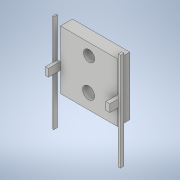
# Autodesk Inventor part: filter wheel
Saved by Autodesk Inventor 2021 (Build 250183000, 183)
## iProperties
Created: 2019-03-06
Part Number: filter wheel
Material: Generic
Document SubType Name: Modeling
Designer: Saumya
Density: 1 g/cm^3
Appearance: Default
Author: Saumya
Autodesk Inventor part; units mm, degrees
ref_plane "YZ Plane" through (0, 0, 0) normal (1, 0, 0) x (0, 1, 0)
ref_plane "XZ Plane" through (0, 0, 0) normal (0, 1, 0) x (-1, 0, 0)
ref_plane "XY Plane" through (0, 0, 0) normal (0, 0, 1) x (1, 0, 0)
sketch "Sketch1" plane through (0, 0, 0) normal (0, 0, 1) x (1, 0, 0)
  circle A0 centre (101.883, 74.9428) radius 12.7
  line L0 (42.2826, 167.437) -> (163.579, 167.437)
  line L1 (163.579, 167.437) -> (163.579, 43.6004)
  line L2 (163.579, 43.6004) -> (42.2826, 43.6004)
  line L3 (42.2826, 43.6004) -> (42.2826, 167.437)
  circle A1 centre (102.9308, 142.9872) radius 11.691
  line L4 (42.2826, 116.6323) -> (31.1691, 116.6323)
  line L5 (31.1691, 116.6323) -> (31.1691, 96.9454)
  line L6 (31.1691, 96.9454) -> (42.2826, 96.9454)
  line L7 (42.2826, 96.9454) -> (42.2826, 116.6323)
  line L8 (163.579, 116.6323) -> (174.375, 116.6323)
  line L9 (174.375, 116.6323) -> (174.375, 96.9454)
  line L10 (174.375, 96.9454) -> (163.579, 96.9454)
  line L11 (163.579, 96.9454) -> (163.579, 116.6323)
  line L12 (31.1691, 126.4757) -> (23.2309, 126.4757)
  line L13 (23.2309, 126.4757) -> (23.2309, 0)
  line L14 (23.2309, 0) -> (31.1691, 0)
  line L15 (31.1691, 0) -> (31.1691, 126.4757)
  line L16 (174.375, 126.4757) -> (184.536, 126.4757)
  line L17 (184.536, 126.4757) -> (184.536, 0)
  line L18 (184.536, 0) -> (174.375, 0)
  line L19 (174.375, 0) -> (174.375, 126.4757)
  point P0 (0, 0)
  dimension "d0" = 25.4
  constraints: 40 end point, 10 parallel, 6 point on line, 5 horizontal, 5 perpendicular, 2 centre point
  measures "d0" diameter of A0
extrude "Extrusion1" add sketch "Sketch1" along normal blind 25.4 contours L0 L1 L2 L3
sketch "Sketch2" plane through (0, 0, 25.4) normal (0, 0, 1) x (1, 0, 0)
  line L0 (42.2826, 167.437) -> (42.2826, 43.6004) projected
  line L1 (42.2826, 102.3361) -> (35.9288, 102.3361)
  line L2 (35.9288, 102.3361) -> (35.9288, 86.2401)
  line L3 (35.9288, 86.2401) -> (42.2826, 86.2401)
  line L4 (42.2826, 86.2401) -> (42.2826, 102.3361)
  line L5 (163.579, 43.6004) -> (163.579, 167.437) projected
  line L6 (163.579, 102.3361) -> (171.9195, 102.3361)
  line L7 (171.9195, 102.3361) -> (171.9195, 86.2401)
  line L8 (171.9195, 86.2401) -> (163.579, 86.2401)
  line L9 (163.579, 86.2401) -> (163.579, 102.3361)
  point P0 (0, 0)
  constraints: 16 end point, 4 parallel, 4 point on line, 2 horizontal, 2 perpendicular
extrude "Extrusion2" add sketch "Sketch2" along normal blind 25.4
sketch "Sketch3" plane through (0, 0, 25.4) normal (0, 0, 1) x (1, 0, 0)
  circle A0 centre (101.883, 74.9428) radius 12.7 projected
  line L0 (35.9288, 184.8101) -> (33.0642, 184.8101)
  line L1 (33.0642, 184.8101) -> (33.0642, -10.6552)
  line L2 (33.0642, -10.6552) -> (35.9288, -10.6552)
  line L3 (35.9288, -10.6552) -> (35.9288, 184.8101)
  line L4 (171.9195, 184.8101) -> (176.5914, 184.8101)
  line L5 (176.5914, 184.8101) -> (176.5914, -10.6552)
  line L6 (176.5914, -10.6552) -> (171.9195, -10.6552)
  line L7 (171.9195, -10.6552) -> (171.9195, 184.8101)
  point P0 (0, 0)
  constraints: 16 end point, 4 parallel, 2 horizontal, 2 perpendicular
extrude "Extrusion3" add sketch "Sketch3" along normal blind 7.62 contours L3 L2 L1 L0 | L4 L5 L6 L7
move faces "Move Face1" translate (0, -11.32, 0) faces at (175.0341, -10.6552, 27.94) (34.0191, -10.6552, 27.94)
body "Solid1"
